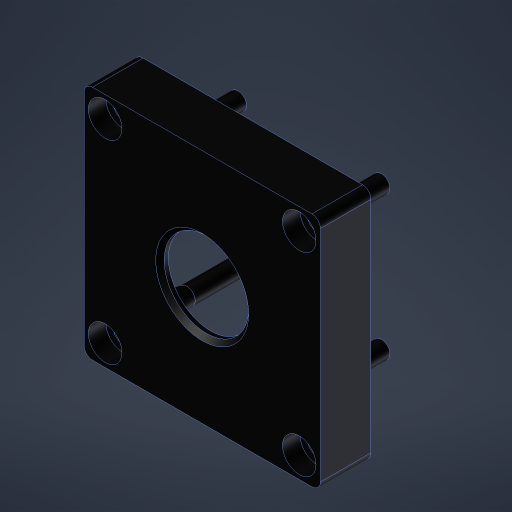
# Autodesk Inventor part: ELP Camera Lid
Saved by Autodesk Inventor 2023 (Build 270158000, 158)
## iProperties
Created: 2024-02-12
Part Number: ELP Camera Lid
Material: Aluminum 6061
Document SubType Name: Modeling
Designer: mavericks
Density: 2.7 g/cm^3
Appearance: Aluminum - Flat
Author: mavericks
Autodesk Inventor part; units mm, degrees
ref_plane "YZ Plane" through (0, 0, 0) normal (1, 0, 0) x (0, 1, 0)
ref_plane "XZ Plane" through (0, 0, 0) normal (0, 1, 0) x (-1, 0, 0)
ref_plane "XY Plane" through (0, 0, 0) normal (0, 0, 1) x (1, 0, 0)
derived "ELP Camera Case.ipt"
sketch "Sketch1" plane through (0, 0, 0) normal (0, 0, 1) x (1, 0, 0)
  line L0 (-19, 19) -> (19, 19) construction
  line L1 (19, 19) -> (19, -19) construction
  line L2 (19, -19) -> (-19, -19) construction
  line L3 (-19, -19) -> (-19, 19) construction
  line L4 (-19, 19) -> (19, -19) construction
  line L5 (19, 19) -> (-19, -19) construction
  line L6 (-17, 17) -> (17, 17) construction
  line L7 (17, 17) -> (17, -17) construction
  line L8 (17, -17) -> (-17, -17) construction
  line L9 (-17, -17) -> (-17, 17) construction
  line L10 (-17, 17) -> (17, -17) construction
  line L11 (17, 17) -> (-17, -17) construction
  line L12 (28, 28) -> (-28, 28)
  line L13 (-28, 28) -> (-28, -28)
  line L14 (-28, -28) -> (28, -28)
  line L15 (28, -28) -> (28, 28)
  circle A0 centre (-23, 23) radius 5 construction
  circle A1 centre (23, 23) radius 5 construction
  line L16 (23, -23) -> (-23, -23) construction
  line L17 (-23, -23) -> (-23, 23) construction
  line L18 (-23, 23) -> (23, 23) construction
  line L19 (23, 23) -> (23, -23) construction
  line L20 (23, -23) -> (-23, 23) construction
  line L21 (-23, -23) -> (23, 23) construction
  circle A2 centre (-17, 17) radius 2
  circle A3 centre (17, 17) radius 2
  circle A4 centre (17, -17) radius 2
  circle A5 centre (-17, -17) radius 2
  point P0 (0, 0)
sketch "Sketch2" plane through (0, 0, 0) normal (0, 0, 1) x (1, 0, 0)
  line L0 (28, 28) -> (-28, 28) projected
  line L1 (28, -28) -> (28, 28) projected
  line L2 (-28, -28) -> (28, -28) projected
  line L3 (-28, 28) -> (-28, -28) projected
  circle A0 centre (-17, -17) radius 2 projected
  circle A1 centre (17, -17) radius 2 projected
  circle A2 centre (17, 17) radius 2 projected
  circle A3 centre (-17, 17) radius 2 projected
  point P0 (0, 0)
  point P1 (-23, -23)
  point P2 (23, -23)
  point P3 (-23, -23)
  point P4 (-23, 23)
  point P5 (-23, 23)
  point P6 (23, 23)
extrude "Extrusion1" add sketch "Sketch2" along normal blind 12 contours L1 L2 L3 L0 | A0 | A1 | A2 | A3
sketch "Sketch6" plane through (0, 0, 12) normal (0, 0, 1) x (1, 0, 0)
  point P0 (0, 0)
  point P1 (23, 23)
  point P2 (-23, 23)
  point P3 (-23, -23)
  point P4 (23, -23)
hole "Hole4" at (23, 23, 12) at (-23, 23, 12) at (-23, -23, 12) at (23, -23, 12) direction (0, 0, -1) diameter 4.496 end through all counterbore diameter 7.938 counterbore depth 4.166 clearance for "Socket Head Cap Screw" size "#8" standard "Ansi Unified Screw Threads"
shell "Shell1" thickness 2 removed faces 1 at (7.1698, -7.1058, 0)
fillet "Fillet1" radius 2 4 edges at (-28, 28, 6) (-28, -28, 6) (28, -28, 6) (28, 28, 6)
extrude "Extrusion2" add sketch "Sketch2" along normal blind 12 and the other way blind 13.5 contours A0 | A1 | A2 | A3
sketch "Sketch3" plane through (17, 17, -13.5) normal (0, 0, -1) x (-1, 0, 0)
  circle A0 centre (0, 0) radius 2 construction
  circle A1 centre (34, 0) radius 2 construction
  circle A2 centre (34, -34) radius 2 construction
  circle A3 centre (0, -34) radius 2 construction
  point P0 (17, -17)
  constraints: 4 coincident
hole "Hole2" at (17, 17, -13.5) at (-17, 17, -13.5) at (-17, -17, -13.5) at (17, -17, -13.5) direction (0, 0, 1) diameter 2.1 depth 2
chamfer "Chamfer1" distance 2 angle 80 4 edges at (15, 17, 10) (-19, 17, 10) (15, -17, 10) (-19, -17, 10) measured on face at (14.5, -17, 10) measured on face at (-19.5, -17, 10) measured on face at (14.5, 17, 10) measured on face at (-19.5, 17, 10)
sketch "Sketch4" plane through (0, 0, 12) normal (0, 0, 1) x (1, 0, 0)
  point P0 (0, 0)
  point P1 (0, 0)
  constraints: 1 coincident
hole "Hole3" at (0, 0, 12) direction (0, 0, -1) diameter 20 end through all
chamfer "Chamfer2" distance 1 angle 45 1 edges at (0, 10, 12)
fillet "Fillet2" radius 1 32 edges at (-26, -17.8397, 7.917) (-23.5414, -17.0556, 10) (-17.0556, -23.5414, 10) (-17.1915, -13.0046, 10) (-14.3102, -19.9606, 10) (-17.8397, -26, 7.917) (-19.9962, -19.9962, 5.834) (-19.9924, -26, 2.917) (-26, -19.9924, 2.917) (-26, 17.8397, 7.917) (-26, 19.9924, 2.917) (-19.9962, 19.9962, 5.834) (-23.5414, 17.0556, 10) (-17.1915, 13.0046, 10) (-14.3102, 19.9606, 10) (-17.0556, 23.5414, 10) (-17.8397, 26, 7.917) (-19.9924, 26, 2.917) (14.0394, 14.3102, 10) (17.0556, 23.5414, 10) (17.8397, 26, 7.917) (19.9924, 26, 2.917) (26, 19.9924, 2.917) (26, 17.8397, 7.917) (23.5414, 17.0556, 10) (14.0394, -14.3102, 10) (23.5414, -17.0556, 10) (26, -17.8397, 7.917) (26, -19.9924, 2.917) (19.9924, -26, 2.917) (17.8397, -26, 7.917) (17.0556, -23.5414, 10)
sketch "Sketch5" plane through (0, 0, 0) normal (1, 0, 0) x (0, 1, 0)
  line L0 (0, 12) -> (0, 150.6963) construction
  line L1 (0, 12) -> (-2665.7407, 1878.5717)
  line L2 (-26, 12) -> (26, 12) projected
  point P0 (0, 0)
  dimension "d36" = 55
  constraints: 4 end point, 1 midpoint, 1 vertical
  measures "d36" angle of L1 L0
body "Solid1"
body "Srf1"
